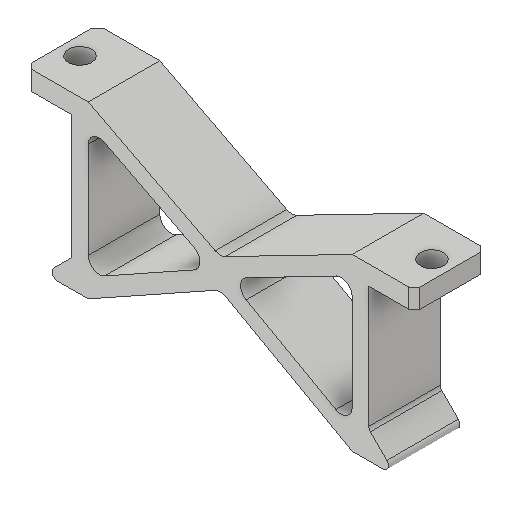
# Autodesk Inventor part: 3DP_PLA_Turbine_stand
Saved by Autodesk Inventor 2026.1 (Build 301233000, 233)
## iProperties
Created: 2020-03-29
Part Number: 3DP_PLA_Turbine_stand
Material: Generic
Document SubType Name: Modeling
Designer: Andrzej
Density: 1 g/cm^3
Appearance: Default
Author: Andrzej
Autodesk Inventor part; units mm, degrees
ref_plane "YZ Plane" through (0, 0, 0) normal (1, 0, 0) x (0, 1, 0)
ref_plane "XZ Plane" through (0, 0, 0) normal (0, 1, 0) x (-1, 0, 0)
ref_plane "XY Plane" through (0, 0, 0) normal (0, 0, 1) x (1, 0, 0)
sketch "Sketch1" plane through (0, 0, 0) normal (0, 0, 1) x (1, 0, 0)
  line L0 (-35.3, 0) -> (-27, 0)
  line L1 (-27, 0) -> (-27, -3.5)
  line L2 (-27, -3.5) -> (-35.3, -3.5)
  line L3 (-35.3, -3.5) -> (-35.3, 0)
  line L4 (-27, 0) -> (-24, 0)
  line L5 (-24, 0) -> (-24, -31)
  line L6 (-24, -31) -> (-27, -31)
  line L7 (-27, -31) -> (-27, 0)
  line L8 (-27, -31) -> (-32, -31)
  line L9 (-32, -31) -> (-27, -26)
  line L10 (-24, -31) -> (36.4267, -31) construction
  line L11 (0, 0) -> (0, -31)
  line L12 (-24, 0) -> (31.066, 0) construction
  line L13 (-24, -31) -> (0, -17.6011)
  line L14 (-24, -27.5641) -> (-1.4552, -14.9777)
  line L15 (-24, 0) -> (0, -12.3526)
  line L16 (-1.4552, -14.9777) -> (-24, -3.374)
  line L17 (35.3, 0) -> (27, 0)
  line L18 (27, 0) -> (27, -3.5)
  line L19 (27, -3.5) -> (35.3, -3.5)
  line L20 (35.3, -3.5) -> (35.3, 0)
  line L21 (27, 0) -> (24, 0)
  line L22 (24, 0) -> (24, -31)
  line L23 (24, -31) -> (27, -31)
  line L24 (27, -31) -> (27, 0)
  line L25 (27, -31) -> (32, -31)
  line L26 (32, -31) -> (27, -26)
  line L27 (24, -31) -> (0, -17.6011)
  line L28 (24, -27.5641) -> (1.4552, -14.9777)
  line L29 (24, 0) -> (0, -12.3526)
  line L30 (1.4552, -14.9777) -> (24, -3.374)
  dimension "d0" = 8.3
  dimension "d1" = 3.5
  dimension "d2" = 27
  dimension "d3" = 3
  dimension "d4" = 31
  dimension "d5" = 5
  dimension "d7" = 45
  dimension "d13" = 0
  dimension "d17" = 3
  dimension "d18" = 3
  constraints: 62 end point, 12 symmetric about line, 9 point on line, 6 parallel, 5 horizontal, 3 perpendicular
  measures "d0" distance of L1.end L2.end
  measures "d1" distance of L0.end L1.end
  measures "d2" distance from line of L11.start L1
  measures "d3" distance of L5.end L6.end
  measures "d4" distance of L4.end L5.end
  measures "d5" distance of L6.end L8.end
  measures "d7" angle of L8 L9
  measures "d13" distance from line of L0 L11.start
  measures "d17" distance between parallel lines of L13 L14
  measures "d18" distance between parallel lines of L15 L16
extrude "Extrusion1" add sketch "Sketch1" along normal blind 13 contours L0 L1 L2 L3 | L4 L5 L6 L7 L1 | L15 L11 L13 L5 L14 L16 | L7 L8 L9 | L29 L22 L30 L28 L27 L11 | L21 L18 L24 L23 L22 | L17 L20 L19 L18 | L24 L26 L25
sketch "Sketch2" plane through (-35.3, 0, 0) normal (0, 1, 0) x (1, 0, 0)
  line L0 (0, 0) -> (11.3, 0) projected
  line L1 (0, 0) -> (0, -13) projected
  line L2 (11.3, -13) -> (0, -13) projected
  line L3 (11.3, 0) -> (11.3, -13) projected
  line L4 (59.3, 0) -> (70.6, 0) projected
  line L5 (59.3, 0) -> (59.3, -13) projected
  line L6 (70.6, -13) -> (59.3, -13) projected
  line L7 (70.6, 0) -> (70.6, -13) projected
  point P0 (35.3, 0)
  point P1 (3.3, -6.5)
  point P2 (67.3, -6.5)
  dimension "d21" = 64
  dimension "d22" = 70.6
  dimension "d23" = 3.3
  dimension "d24" = 6.5
  dimension "d25" = 13
  measures "d21" distance of point (67.3, -6.5) point (3.3, -6.5)
  measures "d22" distance between parallel lines of L7 L1
  measures "d23" distance from line of L1 point (3.3, -6.5)
  measures "d24" distance from line of L2 point (3.3, -6.5)
  measures "d25" distance between parallel lines of L2 L0
hole "Hole1" at (-32, 0, 6.5) at (32, 0, 6.5) direction (0, -1, 0) diameter 4.2 depth 15 tip angle 118
fillet "Fillet1" radius 2 8 edges at (0, -12.3526, 6.5) (0, -17.6011, 6.5) (1.4552, -14.9777, 6.5) (-1.4552, -14.9777, 6.5) (-24, -27.5641, 6.5) (-24, -3.374, 6.5) (24, -3.374, 6.5) (24, -27.5641, 6.5)
fillet "Fillet1" radius 1 4 edges at (-27, -26, 6.5) (-32, -31, 6.5) (27, -26, 6.5) (32, -31, 6.5)
chamfer "Chamfer1" distance 1 angle 45 4 edges at (35.3, -1.75, 13) (35.3, -1.75, 0) (-35.3, -1.75, 0) (-35.3, -1.75, 13)
equation "\"d23\" = -0.5 * d21 + 0.5 * d22"
equation "\"d24\" = 0.5 * d25"
equation "\"d16\" = d12"
equation "\"d12\" = 3"
body "Solid1"
